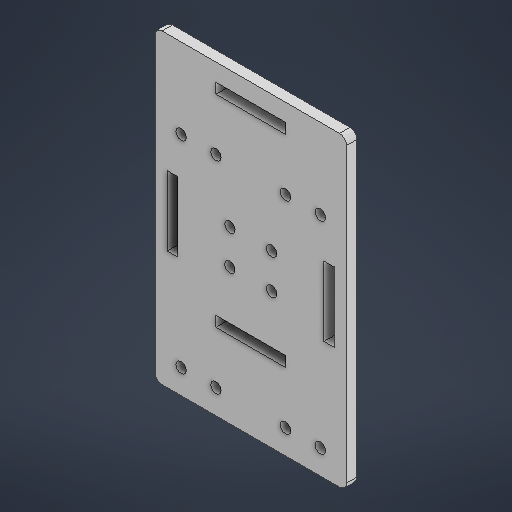
# Autodesk Inventor part: PlacaFrontalSTD
Saved by Autodesk Inventor 2026.2 (Build 302298010, 298A)
## iProperties
Created: 2026-04-16
Part Number: PlacaFrontalSTD
Material: Genérico
Document SubType Name: Modeling
Designer: Jose Carlos
Density: 1 g/cm^3
Appearance: Valor por defecto
Author: Jose Carlos
Autodesk Inventor part; units mm, degrees
ref_plane "YZ Plane" through (0, 0, 0) normal (1, 0, 0) x (0, 1, 0)
ref_plane "XZ Plane" through (0, 0, 0) normal (0, 1, 0) x (-1, 0, 0)
ref_plane "XY Plane" through (0, 0, 0) normal (0, 0, 1) x (1, 0, 0)
sketch "Boceto1" plane through (0, 0, 0) normal (0, 0, 1) x (1, 0, 0)
  line L0 (27.5, -44) -> (-27.5, -44)
  line L1 (-27.5, -44) -> (-27.5, 44)
  line L2 (-27.5, 44) -> (27.5, 44)
  line L3 (27.5, 44) -> (27.5, -44)
  line L4 (27.5, -44) -> (-27.5, 44) construction
  line L5 (-27.5, -44) -> (27.5, 44) construction
  point P0 (0, 0)
  dimension "d0" = 55
  dimension "d1" = 88
  constraints: 12 end point, 2 midpoint, 2 parallel, 1 horizontal, 1 perpendicular
  measures "d0" distance of L1.end L2.end
  measures "d1" distance of L0.end L1.end
extrude "Extrusión1" add sketch "Boceto1" along normal blind 3
sketch "Boceto2" plane through (0, 0, 3) normal (0, 0, 1) x (1, 0, 0)
  line L0 (0, 61.6) -> (0, -61.6) construction
  line L1 (-27.5, -44) -> (27.5, -44) construction
  line L2 (27.5, 44) -> (-27.5, 44) construction
  point P0 (0, 0)
  point P1 (-20, -37)
  point P2 (-10, -37)
  point P3 (20, -37)
  point P4 (10, -37)
  point P5 (-20, 21)
  point P6 (-10, 21)
  point P7 (20, 21)
  point P8 (10, 21)
  dimension "d4" = 10
  dimension "d5" = 0
  dimension "d7" = 10
  dimension "d8" = 7
  dimension "d22" = 23
  dimension "d23" = 10
  dimension "d24" = 0
  dimension "d25" = 10
  constraints: 4 symmetric about line
  measures "d4" distance of point (-10, -37) point (-20, -37)
  measures "d5" vertical distance of point (-20, -37) point (-10, -37)
  measures "d7" distance from line of L0 point (-10, -37)
  measures "d8" distance from line of L1 point (-20, -37)
  measures "d22" distance from line of L2 point (-20, 21)
  measures "d23" distance of point (-10, 21) point (-20, 21)
  measures "d24" vertical distance of point (-20, 21) point (-10, 21)
  measures "d25" distance from line of L0 point (-10, 21)
hole "Agujero1" at (-20, -37, 3) at (-10, -37, 3) at (20, -37, 3) at (10, -37, 3) at (-20, 21, 3) at (-10, 21, 3) at (10, 21, 3) at (20, 21, 3) direction (0, 0, -1) diameter 3 end through all
sketch "Boceto3" plane through (0, 0, 3) normal (0, 0, 1) x (1, 0, 0)
  line L0 (10, -22) -> (-10, -22)
  line L1 (-10, -22) -> (-10, -19)
  line L2 (-10, -19) -> (10, -19)
  line L3 (10, -19) -> (10, -22)
  line L4 (10, -22) -> (-10, -19) construction
  line L5 (-10, -22) -> (10, -19) construction
  line L6 (0, 61.6) -> (0, -61.6) construction
  circle A0 centre (-10, -37) radius 1.5 construction
  line L7 (10, 36) -> (-10, 36)
  line L8 (-10, 36) -> (-10, 39)
  line L9 (-10, 39) -> (10, 39)
  line L10 (10, 39) -> (10, 36)
  line L11 (10, 36) -> (-10, 39) construction
  line L12 (-10, 36) -> (10, 39) construction
  circle A1 centre (-10, 21) radius 1.5 construction
  point P0 (0, 0)
  point P1 (0, -20.5)
  point P2 (0, 37.5)
  point P3 (0, 36)
  dimension "d16" = 3
  dimension "d17" = 20
  dimension "d21" = 15
  dimension "d26" = 3
  dimension "d27" = 20
  dimension "d28" = 15
  constraints: 24 end point, 5 midpoint, 4 parallel, 2 horizontal, 2 perpendicular, 2 point on line
  measures "d16" distance of L0.end L1.end
  measures "d17" distance of L1.end L2.end
  measures "d21" distance from line of L0 A0.centre
  measures "d26" distance of L7.end L8.end
  measures "d27" distance of L8.end L9.end
  measures "d28" vertical distance of A1.centre point (0, 36)
extrude "Extrusión2" cut sketch "Boceto3" against normal through all
fillet "Empalme1" radius 2 4 edges at (-27.5, -44, 1.5) (27.5, -44, 1.5) (27.5, 44, 1.5) (-27.5, 44, 1.5)
sketch "Boceto5" plane through (0, 0, 3) normal (0, 0, 1) x (1, 0, 0)
  circle A0 centre (-6, 5) radius 1.6 construction
  circle A1 centre (-6, -5) radius 1.6 construction
  circle A2 centre (6, -5) radius 1.6 construction
  circle A3 centre (6, 5) radius 1.6 construction
  constraints: 4 centre point, 8 other
hole "Agujero2" at (-6, 5, 3) at (-6, -5, 3) at (6, -5, 3) at (6, 5, 3) direction (0, 0, -1) diameter 3 end through all
sketch "Boceto6" plane through (0, 0, 3) normal (0, 0, 1) x (1, 0, 0)
  line L0 (-21, -10) -> (-24, -10)
  line L1 (-24, -10) -> (-24, 10)
  line L2 (-24, 10) -> (-21, 10)
  line L3 (-21, 10) -> (-21, -10)
  line L4 (-38.5, 0) -> (38.5, 0) construction
  line L5 (0, 61.6) -> (0, -61.6) construction
  line L6 (21, -10) -> (24, -10)
  line L7 (24, -10) -> (24, 10)
  line L8 (24, 10) -> (21, 10)
  line L9 (21, 10) -> (21, -10)
  line L10 (-21, 14) -> (-21, -14) construction
  point P0 (0, 0)
  point P1 (-24, 0)
  point P2 (22, -14)
  point P3 (24, 0)
  dimension "d37" = 20
  dimension "d38" = 3
  constraints: 18 end point, 5 symmetric about line, 2 parallel, 2 point on line, 1 horizontal, 1 midpoint, 1 perpendicular, 1 vertical, 2 other
  measures "d37" distance of L0.end L1.end
  measures "d38" distance of L1.end L2.end
extrude "Extrusión3" cut sketch "Boceto6" against normal through all
